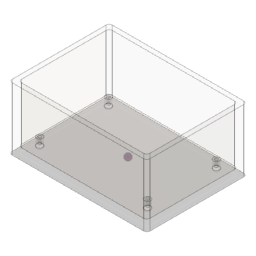
Light project case v1 v3 (Autodesk Fusion 360 design; units mm, degrees)
Autodesk Fusion 360 part; units mm, degrees
sketch "Sketch1" plane through (0, 0, 0) normal (0, 1, 0) x (1, 0, 0) in component "Case"
  line L0 (55.88, 40.64) -> (-55.88, 40.64)
  line L1 (-55.88, 40.64) -> (-55.88, -40.64)
  line L2 (-55.88, -40.64) -> (55.88, -40.64)
  line L3 (55.88, -40.64) -> (55.88, 40.64)
  line L4 (55.88, 40.64) -> (-55.88, -40.64) construction
  line L5 (-55.88, 40.64) -> (55.88, -40.64) construction
  dimension "d2" = 111.76
  dimension "d3" = 81.28
extrude "Extrude1" add sketch "Sketch1" along normal blind 50.8 in component "Case"
sketch "Sketch2" plane through (0, 50.8, 0) normal (0, 1, 0) x (-1, 0, 0) in component "Case"
  line L0 (-55.88, 40.64) -> (-55.88, -40.64)
  line L1 (-55.88, -40.64) -> (55.88, -40.64)
  line L2 (55.88, -40.64) -> (55.88, 40.64)
  line L3 (55.88, 40.64) -> (-55.88, 40.64)
  line L4 (-52.07, -36.83) -> (52.07, -36.83)
  line L5 (52.07, -36.83) -> (52.07, 36.83)
  line L6 (52.07, 36.83) -> (-52.07, 36.83)
  line L7 (-52.07, 36.83) -> (-52.07, -36.83)
  line L8 (-52.07, -36.83) -> (52.07, 36.83) construction
  line L9 (52.07, -36.83) -> (-52.07, 36.83) construction
  dimension "d15" = 3.81
  dimension "d16" = 3.81
  dimension "d17" = 5.08
  dimension "d18" = 5.08
  measures "d15" distance of L2 L5
  measures "d16" distance of L3 L6
  measures "d17" distance of L0 L7
  measures "d18" distance of L1 L4
extrude "Extrude2" cut sketch "Sketch2" against normal blind 45.72 contours L4 L5 L6 L7 in component "Case"
fillet "Fillet1" radius 2.54 1 edges at (-52.07, 27.94, -36.83) in component "Case"
fillet "Fillet2" radius 2.54 3 edges at (52.07, 27.94, 36.83) (52.07, 27.94, -36.83) (-52.07, 27.94, 36.83) in component "Case"
fillet "Fillet3" radius 2.54 4 edges at (55.88, 25.4, -40.64) (55.88, 25.4, 40.64) (-55.88, 25.4, 40.64) (-55.88, 25.4, -40.64) in component "Case"
sketch "Sketch12" plane through (0, 5.08, 0) normal (0, 1, 0) x (-1, 0, 0)
  arc A0 (52.07, 34.29) -> (49.53, 36.83) centre (49.53, 34.29) ccw
  line L0 (49.53, 36.83) -> (-49.53, 36.83)
  arc A1 (-49.53, 36.83) -> (-52.07, 34.29) centre (-49.53, 34.29) ccw
  line L1 (-52.07, 34.29) -> (-52.07, -34.29)
  arc A2 (-52.07, -34.29) -> (-49.53, -36.83) centre (-49.53, -34.29) ccw
  line L2 (-49.53, -36.83) -> (49.53, -36.83)
  arc A3 (49.53, -36.83) -> (52.07, -34.29) centre (49.53, -34.29) ccw
  line L3 (52.07, -34.29) -> (52.07, 34.29)
  line L4 (-43.815, -27.94) -> (43.815, 27.94) construction
  line L5 (43.815, -27.94) -> (-43.815, 27.94) construction
  dimension "d60" = 87.63
  dimension "d61" = 55.88
sketch "Sketch13" plane through (0, 5.08, 0) normal (0, 1, 0) x (-1, 0, 0)
  circle A0 centre (43.815, -27.94) radius 2.54
  circle A1 centre (43.815, 27.94) radius 2.54
  circle A2 centre (-43.815, 27.94) radius 2.54
  circle A3 centre (-43.815, -27.94) radius 2.54
  dimension "d62" = 5.08
  dimension "d63" = 5.08
  dimension "d64" = 5.08
  dimension "d65" = 5.08
  measures "d62" diameter of A0
  measures "d63" diameter of A1
  measures "d64" diameter of A2
  measures "d65" diameter of A3
sketch "Sketch14" plane through (0, 5.08, 0) normal (0, 1, 0) x (-1, 0, 0)
  circle A0 centre (-43.815, -27.94) radius 2.54
  circle A1 centre (-43.815, 27.94) radius 2.54
  circle A2 centre (43.815, 27.94) radius 2.54
  circle A3 centre (43.815, -27.94) radius 2.54
  dimension "d68" = 5.08
  dimension "d69" = 5.08
  dimension "d70" = 5.08
  dimension "d71" = 5.08
  measures "d68" diameter of A0
  measures "d69" diameter of A1
  measures "d70" diameter of A2
  measures "d71" diameter of A3
extrude "Extrude12" add sketch "Sketch14" along normal blind 6.35 contours A0 in component "Case"
sketch "Sketch15" plane through (0, 5.08, 0) normal (0, 1, 0) x (-1, 0, 0)
  circle A0 centre (-43.815, 27.94) radius 2.54
  dimension "d74" = 5.08
  measures "d74" diameter of A0
extrude "Extrude13" add sketch "Sketch15" along normal blind 6.35 in component "Case"
sketch "Sketch16" plane through (0, 5.08, 0) normal (0, 1, 0) x (-1, 0, 0)
  circle A0 centre (43.815, 27.94) radius 2.54
  dimension "d77" = 5.08
  measures "d77" diameter of A0
extrude "Extrude14" add sketch "Sketch16" along normal blind 6.35 in component "Case"
sketch "Sketch17" plane through (0, 5.08, 0) normal (0, 1, 0) x (-1, 0, 0)
  circle A0 centre (43.815, -27.94) radius 2.54
  dimension "d80" = 5.08
  measures "d80" diameter of A0
extrude "Extrude15" add sketch "Sketch17" along normal blind 6.35 in component "Case"
sketch "Sketch18" plane through (-52.07, 0, 0) normal (1, 0, 0) x (0, 0, -1)
  line L0 (-34.29, 50.8) -> (-34.29, 5.08)
  line L1 (-34.29, 5.08) -> (34.29, 5.08)
  line L2 (34.29, 5.08) -> (34.29, 50.8)
  line L3 (34.29, 50.8) -> (-34.29, 50.8)
sketch "Sketch19" plane through (0, 11.43, 0) normal (0, 1, 0) x (-1, 0, 0)
  circle A0 centre (43.815, -27.94) radius 2.54
  circle A1 centre (43.815, -27.94) radius 1.1938
  dimension "d83" = 2.3876
  measures "d83" diameter of A1
extrude "Extrude16" cut sketch "Sketch19" against normal blind 5.08 contours A1 in component "Case"
sketch "Sketch20" plane through (0, 11.43, 0) normal (0, 1, 0) x (-1, 0, 0)
  circle A0 centre (43.815, 27.94) radius 2.54
  circle A1 centre (43.815, 27.94) radius 1.1938
  dimension "d86" = 2.3876
  measures "d86" diameter of A1
extrude "Extrude17" cut sketch "Sketch20" against normal blind 5.08 contours A1 in component "Case"
sketch "Sketch21" plane through (0, 11.43, 0) normal (0, 1, 0) x (-1, 0, 0)
  circle A0 centre (-43.815, -27.94) radius 2.54
  circle A1 centre (-43.815, -27.94) radius 1.1938
  dimension "d89" = 2.3876
  measures "d89" diameter of A1
extrude "Extrude18" cut sketch "Sketch21" against normal blind 5.08 contours A1 in component "Case"
sketch "Sketch22" plane through (0, 11.43, 0) normal (0, 1, 0) x (-1, 0, 0)
  circle A0 centre (-43.815, 27.94) radius 2.54
  circle A1 centre (-43.815, 27.94) radius 1.1513
  dimension "d92" = 2.3027
  measures "d92" diameter of A1
extrude "Extrude19" cut sketch "Sketch22" against normal blind 5.08 contours A1 in component "Case"
component "Case" placed x (1, 0, 0) y (0, 1, 0) z (0, 0, 1) at (0, 0, 0)
component "lid" placed x (1, 0, 0) y (0, 1, 0) z (0, 0, 1) at (0, 0, 0)
